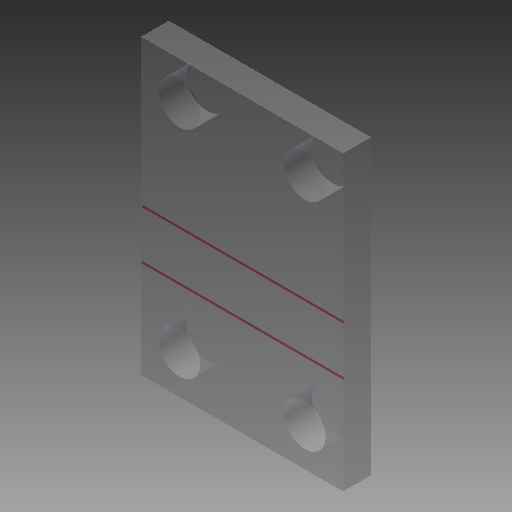
# Autodesk Inventor part: EBARA A Type 馬達側油視窗
Saved by Autodesk Inventor 2018 (Build 220112000, 112)
## iProperties
Created: 2014-01-20
Part Number: EBARA A Type 馬達側油視窗
Material: PMMA 塑膠
Document SubType Name: Modeling
Designer: ERIC
Mass: 5.78794 g
Surface Area: 30.04 cm^2
Volume: 4.872 cm^3
Density: 1.188 g/cm^3
Appearance: 聚碳酸酯 - 透明
Author: ERIC
Autodesk Inventor part; units mm, degrees
ref_plane "YZ Plane" through (0, 0, 0) normal (1, 0, 0) x (0, 1, 0)
ref_plane "XZ Plane" through (0, 0, 0) normal (0, 1, 0) x (-1, 0, 0)
ref_plane "XY Plane" through (0, 0, 0) normal (0, 0, 1) x (1, 0, 0)
sketch "草圖1" plane through (0, 0, 0) normal (0, 0, 1) x (1, 0, 0)
  line L0 (14.5, -21) -> (-14.5, -21)
  line L1 (-14.5, -21) -> (-14.5, 21)
  line L2 (-14.5, 21) -> (14.5, 21)
  line L3 (14.5, 21) -> (14.5, -21)
  line L4 (14.5, 21) -> (-14.5, -21) construction
  point P0 (0, 0)
  dimension "d0" = 29
  dimension "d1" = 42
  constraints: 10 end point, 3 perpendicular, 1 horizontal, 1 midpoint
  measures "d0" distance of L0.start L0.end
  measures "d1" distance of L0.end L1.end
extrude "擠出1" add sketch "草圖1" along normal blind 4
sketch "草圖2" plane through (0, 0, 4) normal (0, 0, 1) x (1, 0, 0)
  line L0 (9, -15.5) -> (-9, -15.5)
  line L1 (-9, -15.5) -> (-9, 15.5)
  line L2 (-9, 15.5) -> (9, 15.5)
  line L3 (9, 15.5) -> (9, -15.5)
  line L4 (9, 15.5) -> (-9, -15.5) construction
  point P0 (0, 0)
  dimension "d4" = 31
  dimension "d5" = 18
  constraints: 10 end point, 3 perpendicular, 1 horizontal, 1 midpoint
  measures "d4" distance of L2.end L0.start
  measures "d5" distance of L1.end L2.end
hole "孔1" at (-9, 15.5, 4) at (9, 15.5, 4) at (9, -15.5, 4) at (-9, -15.5, 4) direction (0, 0, -1) diameter 6 end through all
sketch "草圖3" plane through (0, 0, 4) normal (0, 0, 1) x (1, 0, 0)
  line L0 (-14.5, -21) -> (-14.5, 21) projected
  line L1 (14.5, -21) -> (-14.5, -21) projected
  line L2 (14.5, 21) -> (14.5, -21) projected
  line L3 (-14.5, -6.85) -> (14.5, -6.85)
  line L4 (14.5, -6.85) -> (14.5, -7.15)
  line L5 (14.5, -7.15) -> (-14.5, -7.15)
  line L6 (-14.5, -7.15) -> (-14.5, -6.85)
  line L7 (-14.5, 0.15) -> (14.5, 0.15)
  line L8 (14.5, 0.15) -> (14.5, -0.15)
  line L9 (14.5, -0.15) -> (-14.5, -0.15)
  line L10 (-14.5, -0.15) -> (-14.5, 0.15)
  line L11 (-14.5, -7) -> (14.5, -7)
  line L12 (-14.5, 0) -> (14.5, 0)
  point P0 (0, 0)
  dimension "d13" = 0.3
  dimension "d14" = 0.3
  dimension "d15" = 14
  dimension "d16" = 21
  constraints: 20 end point, 4 midpoint, 4 parallel, 4 point on line, 2 horizontal, 2 perpendicular
  measures "d13" distance between parallel lines of L5 L3
  measures "d14" distance between parallel lines of L9 L7
  measures "d15" distance between parallel lines of L1 L11
  measures "d16" distance between parallel lines of L12 L1
emboss "浮雕1" sketch "草圖3" operation cut depth 0.1 direction (0, 0, -1) contours L0 L11 L2 L5 | L0 L3 L2 L11 | L0 L12 L2 L9 | L0 L7 L2 L12
